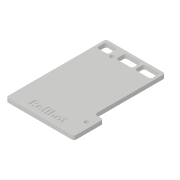
# Autodesk Inventor part: Protective_Plate
Saved by Autodesk Inventor 2019 (Build 230136000, 136)
## iProperties
Created: 2021-06-26
Part Number: Protective_Plate
Material: Generic
Document SubType Name: Modeling
Designer: Oudenas
Density: 1 g/cm^3
Appearance: Default
Author: Oudenas
Autodesk Inventor part; units mm, degrees
ref_plane "YZ Plane" through (0, 0, 0) normal (1, 0, 0) x (0, 1, 0)
ref_plane "XZ Plane" through (0, 0, 0) normal (0, 1, 0) x (-1, 0, 0)
ref_plane "XY Plane" through (0, 0, 0) normal (0, 0, 1) x (1, 0, 0)
sketch "Sketch16" plane through (0, 0, 0) normal (0, 1, 0) x (-1, 0, 0)
  line L0 (25.5, 37.5) -> (-25.5, 37.5)
  line L1 (-25.5, 37.5) -> (-25.5, -37.5)
  line L2 (-25.5, -37.5) -> (25.5, -37.5)
  line L3 (25.5, -37.5) -> (25.5, 37.5)
  line L4 (25.5, 37.5) -> (-25.5, -37.5) construction
  line L5 (-25.5, 37.5) -> (25.5, -37.5) construction
  point P0 (0, 0)
  dimension "d307" = 51
  dimension "d308" = 75
  constraints: 12 end point, 2 midpoint, 2 parallel, 1 horizontal, 1 perpendicular
  measures "d307" distance of L2.end L1.end
  measures "d308" distance of L1.end L0.end
extrude "Extrusion15" add sketch "Sketch16" along normal blind 3
sketch "Sketch17" plane through (0, 3, 0) normal (0, 1, 0) x (1, 0, 0)
  line L0 (25.5, -37.5) -> (25.5, 37.5) projected
  line L1 (25.5, 37.5) -> (19, 37.5)
  line L2 (19, 37.5) -> (19, -15.5)
  line L3 (19, -15.5) -> (25.5, -15.5)
  line L4 (25.5, -15.5) -> (25.5, 37.5)
  point P0 (0, 0)
  dimension "d311" = 6.5
  dimension "d312" = 53
  constraints: 8 end point, 2 parallel, 1 horizontal, 1 perpendicular
  measures "d311" distance of L3.end L2.end
  measures "d312" distance of L2.end L1.end
extrude "Extrusion16" cut sketch "Sketch17" against normal blind 3
sketch "Sketch19" plane through (0, 3, 0) normal (0, 1, 0) x (1, 0, 0)
  circle A0 centre (20.96, -23.53) radius 1.5
  circle A1 centre (15.88, 28.54) radius 1.5
  circle A2 centre (-12.06, 28.54) radius 1.5
  line L0 (25.5, -37.5) -> (25.5, -15.5) projected
  line L1 (-25.5, -37.5) -> (25.5, -37.5) projected
  line L2 (19, -15.5) -> (19, 37.5) projected
  point P0 (0, 0)
  dimension "d315" = 3
  dimension "d316" = 3
  dimension "d317" = 3
  dimension "d319" = 4.54
  dimension "d320" = 13.97
  dimension "d323" = 66.04
  dimension "d324" = 66.04
  dimension "d327" = 9.62
  dimension "d328" = 37.56
  constraints: 3 centre point
  measures "d315" diameter of A0
  measures "d316" diameter of A1
  measures "d317" diameter of A2
  measures "d319" distance from line of L0 A0.centre
  measures "d320" distance from line of L1 A0.centre
  measures "d323" distance from line of A2.centre L1
  measures "d324" distance from line of L1 A1.centre
  measures "d327" distance from line of L0 A1.centre
  measures "d328" distance from line of L0 A2.centre
extrude "Extrusion17" cut sketch "Sketch19" against normal blind 3 contours A0 | A2
sketch "Sketch20" plane through (0, 3, 0) normal (0, 1, 0) x (1, 0, 0)
  line L0 (-9, 35.5) -> (3, 35.5)
  line L1 (3, 35.5) -> (3, 28.5)
  line L2 (3, 28.5) -> (-9, 28.5)
  line L3 (-9, 28.5) -> (-9, 35.5)
  line L4 (19, 37.5) -> (-25.5, 37.5) projected
  line L5 (19, -15.5) -> (19, 37.5) projected
  line L6 (-23.5, 35.5) -> (-15, 35.5)
  line L7 (-15, 35.5) -> (-15, 28.5)
  line L8 (-15, 28.5) -> (-23.5, 28.5)
  line L9 (-23.5, 28.5) -> (-23.5, 35.5)
  line L10 (-25.5, 37.5) -> (-25.5, -37.5) projected
  line L11 (5, 35.5) -> (17, 35.5)
  line L12 (17, 35.5) -> (17, 28.5)
  line L13 (17, 28.5) -> (5, 28.5)
  line L14 (5, 28.5) -> (5, 35.5)
  point P0 (0, 0)
  dimension "d329" = 12
  dimension "d330" = 7
  dimension "d331" = 2
  dimension "d332" = 16
  dimension "d333" = 7
  dimension "d334" = 8.5
  dimension "d335" = 2
  dimension "d336" = 2
  dimension "d343" = 2
  dimension "d344" = 12
  dimension "d345" = 7
  dimension "d346" = 2
  constraints: 24 end point, 6 parallel, 3 horizontal, 3 perpendicular
  measures "d329" distance of L1.end L2.end
  measures "d330" distance of L0.end L1.end
  measures "d331" distance between parallel lines of L0 L4
  measures "d332" distance between parallel lines of L5 L1
  measures "d333" distance between parallel lines of L8 L6
  measures "d334" distance between parallel lines of L7 L9
  measures "d335" distance between parallel lines of L10 L9
  measures "d336" distance between parallel lines of L6 L4
  measures "d343" distance between parallel lines of L4 L11
  measures "d344" distance between parallel lines of L12 L14
  measures "d345" distance between parallel lines of L13 L11
  measures "d346" distance between parallel lines of L5 L12
extrude "Extrusion18" cut sketch "Sketch20" against normal blind 3
fillet "Fillet5" radius 1.5 18 edges at (-23.5, 1.5, -35.5) (-9, 1.5, -35.5) (3, 1.5, -35.5) (-15, 1.5, -35.5) (-23.5, 1.5, -28.5) (-9, 1.5, -28.5) (3, 1.5, -28.5) (-15, 1.5, -28.5) (19, 1.5, -37.5) (-25.5, 1.5, -37.5) (19, 1.5, 15.5) (25.5, 1.5, 15.5) (25.5, 1.5, 37.5) (-25.5, 1.5, 37.5) (5, 1.5, -35.5) (5, 1.5, -28.5) (17, 1.5, -28.5) (17, 1.5, -35.5)
sketch "Sketch18" plane through (0, 3, 0) normal (0, 1, 0) x (1, 0, 0)
  line L0 (-25.4883, -27.714) -> (25.5274, -27.714) construction
  line L1 (25.5274, -27.714) -> (25.5274, -33.7356) construction
  line L2 (25.5274, -33.7356) -> (-25.4883, -33.7356) construction
  line L3 (-25.4883, -33.7356) -> (-25.4883, -27.714) construction
  spline S0 degree 2 poles (-8.53, -33.4928) (-8.53, -33.5393) (-8.5662, -33.6064) (-8.6901, -33.6478) (-8.938, -33.6633) (-9.1497, -33.6633) knots 0 0 0 1 2 3 4 4 4
  spline S1 degree 2 poles (-9.1497, -33.6633) (-9.3253, -33.6633) (-9.537, -33.6478) (-9.661, -33.6013) (-9.7126, -33.529) (-9.7281, -33.4773) knots 0 0 0 1 2 3 4 4 4
  line L4 (-9.7281, -33.4773) -> (-10.2187, -32.2534)
  spline S2 degree 2 poles (-10.2187, -32.2534) (-10.3117, -32.0468) (-10.477, -31.7215) (-10.6887, -31.5046) (-10.9572, -31.3961) (-11.138, -31.3961) knots 0 0 0 1 2 3 4 4 4
  line L5 (-11.138, -31.3961) -> (-11.484, -31.3961)
  line L6 (-11.484, -31.3961) -> (-11.484, -33.4877)
  spline S3 degree 2 poles (-11.484, -33.4877) (-11.484, -33.529) (-11.5408, -33.5961) (-11.6647, -33.6374) (-11.8765, -33.6633) (-12.0417, -33.6633) knots 0 0 0 1 2 3 4 4 4
  spline S4 degree 2 poles (-12.0417, -33.6633) (-12.2018, -33.6633) (-12.4187, -33.6374) (-12.5427, -33.5961) (-12.5943, -33.529) (-12.5943, -33.4877) knots 0 0 0 1 2 3 4 4 4
  line L7 (-12.5943, -33.4877) -> (-12.5943, -28.5144)
  spline S5 degree 2 poles (-12.5943, -28.5144) (-12.5943, -28.3285) (-12.4032, -28.1633) (-12.2638, -28.1633) knots 0 0 0 1 2 2 2
  line L8 (-12.2638, -28.1633) -> (-10.8436, -28.1633)
  spline S6 degree 2 poles (-10.8436, -28.1633) (-10.6319, -28.1633) (-10.353, -28.1787) (-10.2342, -28.1942) knots 0 0 0 1 2 2 2
  spline S7 degree 2 poles (-10.2342, -28.1942) (-9.9037, -28.2407) (-9.377, -28.4679) (-9.0103, -28.8346) (-8.814, -29.3407) (-8.814, -29.6661) knots 0 0 0 1 2 3 4 4 4
  spline S8 degree 2 poles (-8.814, -29.6661) (-8.814, -29.9398) (-8.9535, -30.3891) (-9.2272, -30.7454) (-9.6248, -31.0088) (-9.8779, -31.0863) knots 0 0 0 1 2 3 4 4 4
  spline S9 degree 2 poles (-9.8779, -31.0863) (-9.7539, -31.1482) (-9.537, -31.3187) (-9.346, -31.5562) (-9.1807, -31.8661) (-9.0981, -32.0623) knots 0 0 0 1 2 3 4 4 4
  line L9 (-9.0981, -32.0623) -> (-8.6385, -33.1417)
  spline S10 degree 2 poles (-8.6385, -33.1417) (-8.5713, -33.3018) (-8.53, -33.4515) (-8.53, -33.4928) knots 0 0 0 1 2 2 2
  spline S11 degree 2 poles (-9.9657, -29.7797) (-9.9657, -29.5111) (-10.2136, -29.1393) (-10.4924, -29.0618) knots 0 0 0 1 2 2 2
  spline S12 degree 2 poles (-10.4924, -29.0618) (-10.5751, -29.0412) (-10.792, -29.0154) (-10.9831, -29.0154) knots 0 0 0 1 2 2 2
  line L10 (-10.9831, -29.0154) -> (-11.484, -29.0154)
  line L11 (-11.484, -29.0154) -> (-11.484, -30.5647)
  line L12 (-11.484, -30.5647) -> (-10.9159, -30.5647)
  spline S13 degree 2 poles (-10.9159, -30.5647) (-10.6784, -30.5647) (-10.322, -30.451) (-10.0845, -30.2445) (-9.9657, -29.9553) (-9.9657, -29.7797) knots 0 0 0 1 2 3 4 4 4
  spline S14 degree 2 poles (-4.2901, -31.4942) (-4.2901, -31.6905) (-4.4657, -31.8764) (-4.6154, -31.8764) knots 0 0 0 1 2 2 2
  line L13 (-4.6154, -31.8764) -> (-6.9136, -31.8764)
  spline S15 degree 2 poles (-6.9136, -31.8764) (-6.9136, -32.1191) (-6.8, -32.5116) (-6.5469, -32.7853) (-6.1544, -32.9299) (-5.8807, -32.9299) knots 0 0 0 1 2 3 4 4 4
  spline S16 degree 2 poles (-5.8807, -32.9299) (-5.6018, -32.9299) (-5.1784, -32.8473) (-4.8685, -32.7543) (-4.6671, -32.6717) (-4.6, -32.6717) knots 0 0 0 1 2 3 4 4 4
  spline S17 degree 2 poles (-4.6, -32.6717) (-4.5638, -32.6717) (-4.5122, -32.7027) (-4.476, -32.775) (-4.4657, -32.9144) (-4.4657, -33.0229) knots 0 0 0 1 2 3 4 4 4
  spline S18 degree 2 poles (-4.4657, -33.0229) (-4.4657, -33.1158) (-4.476, -33.2449) (-4.4915, -33.3379) (-4.5225, -33.405) (-4.5793, -33.4618) (-4.8272, -33.5651) (-5.2093, -33.6633) (-5.7, -33.7356) (-5.9788, -33.7356) knots 0 0 0 1 2 3 4 5 6 7 8 8 8
  spline S19 degree 2 poles (-5.9788, -33.7356) (-6.4798, -33.7356) (-7.2389, -33.4825) (-7.7502, -32.9661) (-7.9981, -32.1811) (-7.9981, -31.6492) knots 0 0 0 1 2 3 4 4 4
  spline S20 degree 2 poles (-7.9981, -31.6492) (-7.9981, -31.1482) (-7.7347, -30.3374) (-7.2338, -29.7745) (-6.5211, -29.4802) (-6.0718, -29.4802) knots 0 0 0 1 2 3 4 4 4
  spline S21 degree 2 poles (-6.0718, -29.4802) (-5.5967, -29.4802) (-4.9253, -29.759) (-4.4915, -30.2548) (-4.2901, -30.9313) (-4.2901, -31.329) knots 0 0 0 1 2 3 4 4 4
  line L14 (-4.2901, -31.329) -> (-4.2901, -31.4942)
  spline S22 degree 2 poles (-5.323, -31.1895) (-5.3126, -30.7454) (-5.6948, -30.2341) (-6.0976, -30.2341) knots 0 0 0 1 2 2 2
  spline S23 degree 2 poles (-6.0976, -30.2341) (-6.299, -30.2341) (-6.5985, -30.3839) (-6.8, -30.6421) (-6.9032, -30.9933) (-6.9136, -31.1895) knots 0 0 0 1 2 3 4 4 4
  line L15 (-6.9136, -31.1895) -> (-5.323, -31.1895)
  spline S24 degree 2 poles (-1.1399, -28.282) (-1.1399, -28.406) (-1.1554, -28.5557) (-1.1915, -28.6332) (-1.2328, -28.6642) (-1.2586, -28.6642) knots 0 0 0 1 2 3 4 4 4
  spline S25 degree 2 poles (-1.2586, -28.6642) (-1.2896, -28.6642) (-1.3619, -28.6332) (-1.4652, -28.6022) (-1.6098, -28.5712) (-1.7079, -28.5712) knots 0 0 0 1 2 3 4 4 4
  spline S26 degree 2 poles (-1.7079, -28.5712) (-1.8216, -28.5712) (-1.9868, -28.6435) (-2.0953, -28.7985) (-2.1469, -29.0464) (-2.1469, -29.2271) knots 0 0 0 1 2 3 4 4 4
  line L16 (-2.1469, -29.2271) -> (-2.1469, -29.5731)
  line L17 (-2.1469, -29.5731) -> (-1.4549, -29.5731)
  spline S27 degree 2 poles (-1.4549, -29.5731) (-1.4187, -29.5731) (-1.3516, -29.6144) (-1.3103, -29.7126) (-1.2896, -29.883) (-1.2896, -30.0018) knots 0 0 0 1 2 3 4 4 4
  spline S28 degree 2 poles (-1.2896, -30.0018) (-1.2896, -30.2393) (-1.3723, -30.4356) (-1.4549, -30.4356) knots 0 0 0 1 2 2 2
  line L18 (-1.4549, -30.4356) -> (-2.1469, -30.4356)
  line L19 (-2.1469, -30.4356) -> (-2.1469, -33.4928)
  spline S29 degree 2 poles (-2.1469, -33.4928) (-2.1469, -33.5341) (-2.1985, -33.6013) (-2.3173, -33.6426) (-2.5291, -33.6633) (-2.6788, -33.6633) knots 0 0 0 1 2 3 4 4 4
  spline S30 degree 2 poles (-2.6788, -33.6633) (-2.8338, -33.6633) (-3.0403, -33.6426) (-3.1643, -33.6013) (-3.2108, -33.5341) (-3.2108, -33.4928) knots 0 0 0 1 2 3 4 4 4
  line L20 (-3.2108, -33.4928) -> (-3.2108, -30.4356)
  line L21 (-3.2108, -30.4356) -> (-3.6859, -30.4356)
  spline S31 degree 2 poles (-3.6859, -30.4356) (-3.7633, -30.4356) (-3.846, -30.2393) (-3.846, -30.0018) knots 0 0 0 1 2 2 2
  spline S32 degree 2 poles (-3.846, -30.0018) (-3.846, -29.883) (-3.8253, -29.7126) (-3.7892, -29.6144) (-3.722, -29.5731) (-3.6807, -29.5731) knots 0 0 0 1 2 3 4 4 4
  line L22 (-3.6807, -29.5731) -> (-3.2108, -29.5731)
  line L23 (-3.2108, -29.5731) -> (-3.2108, -29.2581)
  spline S33 degree 2 poles (-3.2108, -29.2581) (-3.2108, -28.8708) (-3.0558, -28.2924) (-2.7305, -27.9102) (-2.2295, -27.714) (-1.8835, -27.714) knots 0 0 0 1 2 3 4 4 4
  spline S34 degree 2 poles (-1.8835, -27.714) (-1.7183, -27.714) (-1.4239, -27.7708) (-1.2535, -27.8327) (-1.1967, -27.8895) (-1.1554, -27.9928) (-1.1399, -28.1581) (-1.1399, -28.282) knots 0 0 0 1 2 3 4 5 6 6 6
  spline S35 degree 2 poles (0.3888, -33.4928) (0.3888, -33.5341) (0.3371, -33.6013) (0.2132, -33.6426) (0.0118, -33.6633) (-0.1431, -33.6633) knots 0 0 0 1 2 3 4 4 4
  spline S36 degree 2 poles (-0.1431, -33.6633) (-0.2981, -33.6633) (-0.4995, -33.6426) (-0.6234, -33.6013) (-0.6751, -33.5341) (-0.6751, -33.4928) knots 0 0 0 1 2 3 4 4 4
  line L24 (-0.6751, -33.4928) -> (-0.6751, -29.728)
  spline S37 degree 2 poles (-0.6751, -29.728) (-0.6751, -29.6867) (-0.6234, -29.6248) (-0.4995, -29.5783) (-0.2981, -29.5525) (-0.1431, -29.5525) knots 0 0 0 1 2 3 4 4 4
  spline S38 degree 2 poles (-0.1431, -29.5525) (0.0118, -29.5525) (0.2132, -29.5783) (0.3371, -29.6248) (0.3888, -29.6867) (0.3888, -29.728) knots 0 0 0 1 2 3 4 4 4
  line L25 (0.3888, -29.728) -> (0.3888, -33.4928)
  spline S39 degree 2 poles (0.4714, -28.4421) (0.4714, -28.7675) (0.208, -29.0102) (-0.1483, -29.0102) knots 0 0 0 1 2 2 2
  spline S40 degree 2 poles (-0.1483, -29.0102) (-0.5098, -29.0102) (-0.7577, -28.7726) (-0.7577, -28.4628) knots 0 0 0 1 2 2 2
  spline S41 degree 2 poles (-0.7577, -28.4628) (-0.7577, -28.1426) (-0.4995, -27.8947) (-0.138, -27.8947) knots 0 0 0 1 2 2 2
  spline S42 degree 2 poles (-0.138, -27.8947) (0.2184, -27.8947) (0.4714, -28.1374) (0.4714, -28.4421) knots 0 0 0 1 2 2 2
  spline S43 degree 2 poles (5.2536, -31.5562) (5.2536, -32.0623) (5.0315, -32.8628) (4.6184, -33.4309) (4.0141, -33.7356) (3.6268, -33.7356) knots 0 0 0 1 2 3 4 4 4
  spline S44 degree 2 poles (3.6268, -33.7356) (3.4357, -33.7356) (3.1052, -33.6633) (2.8057, -33.5032) (2.5113, -33.2553) (2.3615, -33.0849) knots 0 0 0 1 2 3 4 4 4
  line L26 (2.3615, -33.0849) -> (2.3615, -33.4928)
  spline S45 degree 2 poles (2.3615, -33.4928) (2.3615, -33.5393) (2.3151, -33.6064) (2.2066, -33.6478) (2.031, -33.6633) (1.9019, -33.6633) knots 0 0 0 1 2 3 4 4 4
  spline S46 degree 2 poles (1.9019, -33.6633) (1.7728, -33.6633) (1.6024, -33.6478) (1.4939, -33.6064) (1.4526, -33.5393) (1.4526, -33.4928) knots 0 0 0 1 2 3 4 4 4
  line L27 (1.4526, -33.4928) -> (1.4526, -27.9257)
  spline S47 degree 2 poles (1.4526, -27.9257) (1.4526, -27.8844) (1.5043, -27.8172) (1.6282, -27.7708) (1.8296, -27.7449) (1.9846, -27.7449) knots 0 0 0 1 2 3 4 4 4
  spline S48 degree 2 poles (1.9846, -27.7449) (2.1395, -27.7449) (2.3409, -27.7708) (2.4648, -27.8172) (2.5165, -27.8844) (2.5165, -27.9257) knots 0 0 0 1 2 3 4 4 4
  line L28 (2.5165, -27.9257) -> (2.5165, -30.0172)
  spline S49 degree 2 poles (2.5165, -30.0172) (2.6611, -29.8726) (2.9503, -29.6712) (3.2343, -29.537) (3.5442, -29.4802) (3.7094, -29.4802) knots 0 0 0 1 2 3 4 4 4
  spline S50 degree 2 poles (3.7094, -29.4802) (4.1329, -29.4802) (4.7165, -29.8158) (5.0831, -30.3787) (5.2536, -31.1379) (5.2536, -31.5562) knots 0 0 0 1 2 3 4 4 4
  spline S51 degree 2 poles (4.1484, -31.6337) (4.1484, -31.391) (4.0761, -30.9417) (3.9005, -30.5956) (3.6165, -30.3891) (3.3996, -30.3891) knots 0 0 0 1 2 3 4 4 4
  spline S52 degree 2 poles (3.3996, -30.3891) (3.2911, -30.3891) (3.0897, -30.4459) (2.8728, -30.5905) (2.6456, -30.8229) (2.5165, -30.9881) knots 0 0 0 1 2 3 4 4 4
  line L29 (2.5165, -30.9881) -> (2.5165, -32.2431)
  spline S53 degree 2 poles (2.5165, -32.2431) (2.7437, -32.5323) (3.1517, -32.8318) (3.3789, -32.8318) knots 0 0 0 1 2 2 2
  spline S54 degree 2 poles (3.3789, -32.8318) (3.5855, -32.8318) (3.8747, -32.6201) (4.0658, -32.2792) (4.1484, -31.8506) (4.1484, -31.6337) knots 0 0 0 1 2 3 4 4 4
  spline S55 degree 2 poles (9.9169, -31.5717) (9.9169, -32.052) (9.6639, -32.8473) (9.1475, -33.4205) (8.3676, -33.7356) (7.8461, -33.7356) knots 0 0 0 1 2 3 4 4 4
  spline S56 degree 2 poles (7.8461, -33.7356) (7.3451, -33.7356) (6.6015, -33.4567) (6.1108, -32.9248) (5.8733, -32.1449) (5.8733, -31.644) knots 0 0 0 1 2 3 4 4 4
  spline S57 degree 2 poles (5.8733, -31.644) (5.8733, -31.1637) (6.1315, -30.3633) (6.6479, -29.7952) (7.4226, -29.4802) (7.9442, -29.4802) knots 0 0 0 1 2 3 4 4 4
  spline S58 degree 2 poles (7.9442, -29.4802) (8.4503, -29.4802) (9.1939, -29.7539) (9.6794, -30.2858) (9.9169, -31.0656) (9.9169, -31.5717) knots 0 0 0 1 2 3 4 4 4
  spline S59 degree 2 poles (8.8221, -31.613) (8.8221, -31.3341) (8.7343, -30.8642) (8.5226, -30.5182) (8.1714, -30.3219) (7.9029, -30.3219) knots 0 0 0 1 2 3 4 4 4
  spline S60 degree 2 poles (7.9029, -30.3219) (7.6653, -30.3219) (7.309, -30.4975) (7.0817, -30.828) (6.9681, -31.298) (6.9681, -31.5975) knots 0 0 0 1 2 3 4 4 4
  spline S61 degree 2 poles (6.9681, -31.5975) (6.9681, -31.8764) (7.0611, -32.3464) (7.2676, -32.6924) (7.624, -32.8834) (7.8874, -32.8834) knots 0 0 0 1 2 3 4 4 4
  spline S62 degree 2 poles (7.8874, -32.8834) (8.1301, -32.8834) (8.4813, -32.7079) (8.7137, -32.3825) (8.8221, -31.9126) (8.8221, -31.613) knots 0 0 0 1 2 3 4 4 4
  spline S63 degree 2 poles (12.9949, -33.121) (12.9949, -33.3069) (12.9484, -33.5032) (12.8709, -33.5858) (12.7212, -33.6478) (12.5249, -33.6942) (12.2925, -33.7201) (12.1738, -33.7201) knots 0 0 0 1 2 3 4 5 6 6 6
  spline S64 degree 2 poles (12.1738, -33.7201) (11.8536, -33.7201) (11.3888, -33.56) (11.0841, -33.2243) (10.9395, -32.7182) (10.9395, -32.3722) knots 0 0 0 1 2 3 4 4 4
  line L30 (10.9395, -32.3722) -> (10.9395, -30.4356)
  line L31 (10.9395, -30.4356) -> (10.4902, -30.4356)
  spline S65 degree 2 poles (10.4902, -30.4356) (10.4076, -30.4356) (10.3249, -30.2393) (10.3249, -30.0018) knots 0 0 0 1 2 2 2
  spline S66 degree 2 poles (10.3249, -30.0018) (10.3249, -29.883) (10.3456, -29.7126) (10.3869, -29.6144) (10.4489, -29.5731) (10.4953, -29.5731) knots 0 0 0 1 2 3 4 4 4
  line L32 (10.4953, -29.5731) -> (10.9395, -29.5731)
  line L33 (10.9395, -29.5731) -> (10.9395, -28.7313)
  spline S67 degree 2 poles (10.9395, -28.7313) (10.9395, -28.69) (10.986, -28.6229) (11.1099, -28.5764) (11.3165, -28.5557) (11.4714, -28.5557) knots 0 0 0 1 2 3 4 4 4
  spline S68 degree 2 poles (11.4714, -28.5557) (11.6263, -28.5557) (11.8329, -28.5764) (11.9517, -28.6229) (12.0033, -28.69) (12.0033, -28.7313) knots 0 0 0 1 2 3 4 4 4
  line L34 (12.0033, -28.7313) -> (12.0033, -29.5731)
  line L35 (12.0033, -29.5731) -> (12.8245, -29.5731)
  spline S69 degree 2 poles (12.8245, -29.5731) (12.8658, -29.5731) (12.9329, -29.6144) (12.9742, -29.7126) (12.9949, -29.883) (12.9949, -30.0018) knots 0 0 0 1 2 3 4 4 4
  spline S70 degree 2 poles (12.9949, -30.0018) (12.9949, -30.2393) (12.9123, -30.4356) (12.8296, -30.4356) knots 0 0 0 1 2 2 2
  line L36 (12.8296, -30.4356) -> (12.0033, -30.4356)
  line L37 (12.0033, -30.4356) -> (12.0033, -32.2069)
  spline S71 degree 2 poles (12.0033, -32.2069) (12.0033, -32.5168) (12.1996, -32.8266) (12.4475, -32.8266) knots 0 0 0 1 2 2 2
  spline S72 degree 2 poles (12.4475, -32.8266) (12.5353, -32.8266) (12.6695, -32.7956) (12.7728, -32.7595) (12.8451, -32.7285) (12.8761, -32.7285) knots 0 0 0 1 2 3 4 4 4
  spline S73 degree 2 poles (12.8761, -32.7285) (12.9019, -32.7285) (12.9484, -32.7595) (12.9742, -32.8473) (12.9949, -33.0022) (12.9949, -33.121) knots 0 0 0 1 2 3 4 4 4
  point P0 (0, 0)
  constraints: 2 other
extrude "Extrusion19" cut sketch "Sketch18" against normal blind 0.6
fillet "Fillet6" radius 0.4 19 edges at (-6.9136, 2.7, 31.1895) (-5.323, 2.7, 31.1895) (-6.9136, 2.7, 31.8764) (-11.484, 2.7, 29.0154) (-11.484, 2.7, 30.5647) (-11.484, 2.7, 31.3961) (-9.8779, 2.7, 31.0863) (-2.1469, 2.7, 29.5731) (-3.2108, 2.7, 29.5731) (-3.2108, 2.7, 30.4356) (-2.1469, 2.7, 30.4356) (2.5165, 2.7, 30.0172) (2.3615, 2.7, 33.0849) (2.5165, 2.7, 32.2431) (2.5165, 2.7, 30.9881) (12.0033, 2.7, 29.5731) (10.9395, 2.7, 29.5731) (10.9395, 2.7, 30.4356) (12.0033, 2.7, 30.4356)
body "Solid2"
